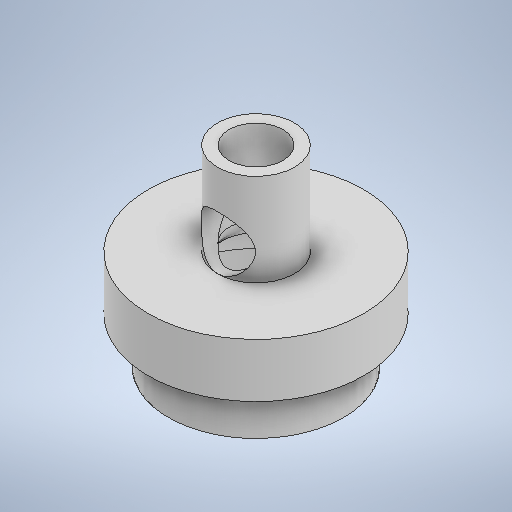
# Autodesk Inventor part: vial_adapter_female
Saved by Autodesk Inventor 2025 (Build 290162010, 162A)
## iProperties
Created: 2023-04-28
Part Number: vial_adapter_female
Material: Generic
Document SubType Name: Modeling
Designer: dinesh
Density: 1 g/cm^3
Appearance: Default
Author: dinesh
Autodesk Inventor part; units mm, degrees
ref_plane "YZ Plane" through (0, 0, 0) normal (1, 0, 0) x (0, 1, 0)
ref_plane "XZ Plane" through (0, 0, 0) normal (0, 1, 0) x (-1, 0, 0)
ref_plane "XY Plane" through (0, 0, 0) normal (0, 0, 1) x (1, 0, 0)
sketch "Sketch1" plane through (0, 0, 0) normal (0, 0, 1) x (1, 0, 0)
  line L0 (3, 13) -> (5, 13)
  line L1 (5, 13) -> (5, 1)
  line L2 (8.5, 0) -> (3.5, 0)
  line L3 (3.5, 2) -> (3.5, 13)
  line L4 (0, 50) -> (0, -50)
  line L5 (3.5, 13) -> (3, 13)
  line L6 (5, 1) -> (14, 1)
  line L7 (14, 1) -> (14, 0)
  line L8 (13, 0) -> (5, 0)
  line L9 (5, 0) -> (5, 1) construction
  line L10 (14, 0) -> (13, 0) construction
  line L11 (13, 0) -> (13, -6)
  line L12 (13, -6) -> (14, -6)
  line L13 (14, -6) -> (14, 0)
  line L14 (11.5, 0) -> (10.5, 0)
  arc A0 (3.5, 2) -> (5.5, 0) centre (5.5, 2) ccw
  line L15 (-4.4, 0) -> (4.4, 0) construction
  line L16 (10.4, 0) -> (11.4, 0)
  line L17 (11.4, 0) -> (11.4, -6)
  line L18 (11.4, -6) -> (10.4, -6) construction
  line L19 (10.4, -6) -> (10.4, -6)
  arc A1 (10.4, -6) -> (4.4, 0) centre (4.4, -6) ccw
  line L20 (11.4, -6) -> (11.4, -12)
  line L21 (11.4, -12) -> (11.3, -12)
  line L22 (11.3, -12) -> (10.4, -6)
  point P0 (0, 0)
  point P1 (11.4, 0)
  point P2 (5.5, 0)
  point P3 (4.4, 0)
  dimension "d0" = 7
  dimension "d1" = 13
  dimension "d2" = 10
  dimension "d5" = 1
  dimension "d6" = 26
  dimension "d7" = 1
  dimension "d8" = 6
  dimension "d11" = 2
  dimension "d12" = 100
  dimension "d15" = 1
  dimension "d16" = 1.6
  dimension "d17" = 6
  dimension "d27" = 0.1
  dimension "d28" = 6
  constraints: 46 end point, 8 parallel, 7 horizontal, 5 perpendicular, 4 point on circle, 4 point on line, 4 tangent, 3 collinear, 3 midpoint, 2 centre point, 2 vertical
  measures "d0" diameter of L3 L4
  measures "d1" distance between parallel lines of L0 L2
  measures "d2" diameter of L1 L4
  measures "d5" distance between parallel lines of L8 L6
  measures "d6" diameter of L11 L4
  measures "d7" distance between parallel lines of L11 L13
  measures "d8" distance between parallel lines of L12 L8
  measures "d11" radius of A0
  measures "d12" distance of L4.start L4.end
  measures "d15" distance between parallel lines of L17 L19
  measures "d16" distance between parallel lines of L11 L17
  measures "d17" radius of A1
  measures "d27" distance of L20.end L21.end
  measures "d28" distance of L17.end L20.end
revolve "Revolution1" add sketch "Sketch1" angle 360 about axis through (0, 50, 0) along (0, -1, 0)
sketch "Sketch2" plane through (0, 0, 0) normal (0, 0, 1) x (1, 0, 0)
  line L0 (-3.5, 2) -> (3.5, 2) construction
  circle A0 centre (0, 4.5) radius 3.5
  line L1 (-5.5, 0) -> (5.5, 0) projected
  line L2 (-5, 13) -> (5, 13) projected
  line L3 (0, 13) -> (0, 0) construction
  point P0 (2.4495, 2)
  point P1 (-2.4495, 2)
  dimension "d1" = 13
  dimension "d19" = 7
  dimension "d26" = 4.5
  constraints: 2 end point, 1 centre point, 1 midpoint, 1 point on line, 1 vertical
  measures "d19" diameter of A0
  measures "d26" distance from line of A0.centre L1
extrude "Extrusion1" cut sketch "Sketch2" along normal blind 10 and the other way blind 3.1
equation "\"d0\" = t_D_f"
equation "\"d1\" = top_th_f + w_th"
equation "\"d2\" = top_D"
equation "\"d5\" = w_th"
equation "\"d6\" = lv_OD"
equation "\"d7\" = w_th"
equation "\"d8\" = w_l"
equation "\"d11\" = fillet_D"
equation "\"d15\" = w_th"
equation "\"d16\" = lv_th"
equation "\"d17\" = 3 * fillet_D"
equation "\"d27\" = tol"
equation "\"d28\" = w_l"
equation "\"d19\" = t_D_f"
equation "\"d26\" = 0.5 * t_D_f + w_th"
equation "\"d21\" = top_D"
equation "\"d22\" = 0.5 * t_D + tol"
equation "\"tol\" = 0.1"
equation "\"fillet_D\" = 2"
equation "\"w_th\" = 1"
equation "\"w_l\" = 6"
equation "\"t_D\" = 6"
equation "\"top_D\" = 10"
equation "\"cn_h\" = 5"
equation "\"lv_OD\" = 26"
equation "\"lv_th\" = 1.6"
equation "\"t_D_f\" = t_D + w_th"
equation "\"top_th_f\" = t_D_f + cn_h"
equation "\"top_th\" = t_D + w_th"
equation "\"sv_OD\" = 13"
equation "\"sv_th\" = 1.5"
equation "\"b_OD\" = 44"
equation "\"b_th\" = 1.5"
equation "\"b_ID\" = 36.5"
equation "\"b_rim_h\" = 5"
equation "\"h_D\" = 0.9"
equation "\"h_s\" = 2.25"
equation "\"v_h_D\" = 7.5"
equation "\"v_h_off\" = 0.5 * cn_D + 0.5 * v_h_D"
equation "\"cn_D\" = 13.2"
body "Solid1"
